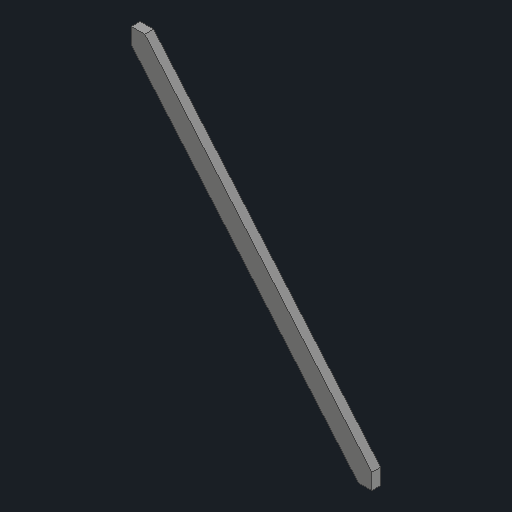
# Autodesk Inventor part: 2x4x44
Saved by Autodesk Inventor 2026 (Build 300175000, 175)
## iProperties
Created: 2024-09-20
Part Number: 2x4x44
Material: Generic
Document SubType Name: Modeling
Designer: User
Density: 1 g/cm^3
Appearance: Default
Finish1_Area: 623.223 in^2
Finish1_Appearance: Red
Finish1_Process: Prime/Paint RAL 3018
Finish1_Description: Prime/Paint RAL 3018
Finish1_ShortDescription: RAL 3018
Finish1_Thickness: 0.002 in
Author: User
Autodesk Inventor part; units mm, degrees
ref_plane "YZ Plane" through (0, 0, 0) normal (1, 0, 0) x (0, 1, 0)
ref_plane "XZ Plane" through (0, 0, 0) normal (0, 1, 0) x (-1, 0, 0)
ref_plane "XY Plane" through (0, 0, 0) normal (0, 0, 1) x (1, 0, 0)
sketch "Sketch1" plane through (0, 0, 0) normal (0, 0, 1) x (1, 0, 0)
  line L0 (-1041.4, 1219.2) -> (-1041.4, 0) projected
  line L1 (-1041.4, 1219.2) -> (0, 1219.2) projected
  line L2 (0, 0) -> (0, 1219.2) projected
  line L3 (0, 0) -> (-1041.4, 0) projected
  line L4 (0, 0) -> (0, 68.4388)
  line L5 (0, 68.4388) -> (-982.9419, 1219.2)
  line L6 (-982.9419, 1219.2) -> (-1041.4, 1219.2)
  line L7 (-1041.4, 1219.2) -> (-1041.4, 1150.7612)
  line L8 (-1041.4, 1150.7612) -> (-58.4581, 0)
  line L9 (-58.4581, 0) -> (0, 0)
  constraints: 12 end point, 4 point on line, 2 collinear, 1 parallel
extrude "Extrusion1" add sketch "Sketch1" against normal blind 38.1 contours L1 L5 L2 L3 L8 L0
body "Solid1"
